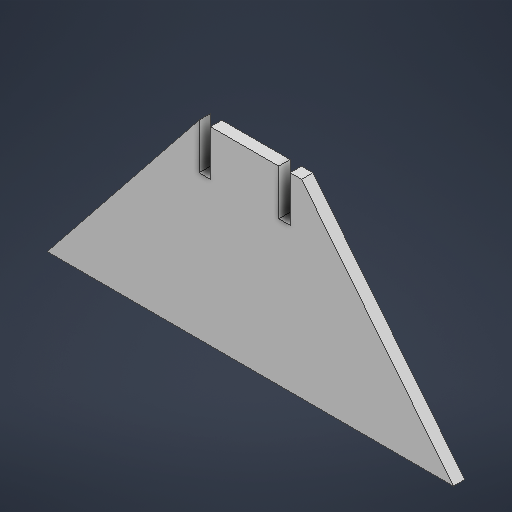
# Autodesk Inventor part: Base
Saved by Autodesk Inventor 2027 (Build 310192000, 192)
## iProperties
Created: 2026-05-24
Part Number: Base
Material: Generic
Document SubType Name: Modeling
Designer: alexy
Density: 1 g/cm^3
Appearance: Default
Author: alexy
Autodesk Inventor part; units mm, degrees
ref_plane "YZ Plane" through (0, 0, 0) normal (1, 0, 0) x (0, 1, 0)
ref_plane "XZ Plane" through (0, 0, 0) normal (0, 1, 0) x (-1, 0, 0)
ref_plane "XY Plane" through (0, 0, 0) normal (0, 0, 1) x (1, 0, 0)
sketch "Sketch1" plane through (0, 0, 0) normal (0, 0, 1) x (1, 0, 0)
  line L0 (0, 0) -> (0, 12)
  line L1 (0, 12) -> (0, 12)
  line L2 (0, 12) -> (0, 0)
  line L3 (0, 0) -> (3, 0)
  line L4 (3, 0) -> (3, 12)
  line L5 (3, 12) -> (6, 12)
  line L6 (6, 12) -> (46, -38)
  line L7 (46, -38) -> (-61, -38)
  line L8 (0, 12) -> (-18, 12)
  line L9 (-18, 12) -> (-18, 0)
  line L10 (-18, 0) -> (-21, 0)
  line L11 (-21, 0) -> (-21, 12)
  line L12 (-21, 12) -> (-61, -38)
  point P0 (1.5, 0)
  dimension "d0" = 3
  dimension "d1" = 12
  dimension "d2" = 3
  dimension "d3" = 18
  dimension "d8" = 3
  dimension "d9" = 40
  dimension "d10" = 40
  dimension "d11" = 50
  constraints: 26 end point, 6 perpendicular, 2 horizontal alignment, 2 point on line, 2 vertical, 1 coincident, 1 horizontal, 1 midpoint, 1 parallel, 1 vertical alignment
  measures "d0" distance of L2.end L3.end
  measures "d1" distance of L3.end L4.end
  measures "d2" distance of L4.end L5.end
  measures "d3" distance of L1.end L8.end
  measures "d8" distance of L9.end L10.end
  measures "d9" horizontal distance of L7.end L11.end
  measures "d10" horizontal distance of L6.end L5.end
  measures "d11" vertical distance of L6.end L5.end
extrude "Extrusion1" add sketch "Sketch1" along normal blind 3
body "Solid1"
